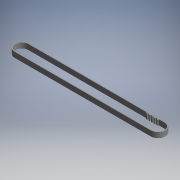
# Autodesk Inventor part: HTBN600S5M-100_info-1-16-16
Saved by Autodesk Inventor 2017.3 (Build 213256000, 256)
## iProperties
Part Number: HTBN600S5M-100_info-1-16-16
Material: Generic
Catalog Web Link: www.cadenas.de
Description: HTBN__S5M-High TorqueTiming Belts S5M (Pitch 5mm)
Vendor: MISUMI
Document SubType Name: Modeling
Designer: partserver
Manufacturer: MISUMI
Mass: 9.29796 g
Surface Area: 140.356 cm^2
Volume: 9.29796 cm^3
Density: 1 g/cm^3
Appearance: PSOLRGB-175-175-175
Category: PARTsolutions
Company: MISUMI
Title: HTBN600S5M-100
Author: Cadenas PARTsolutions
Comments: High TorqueTiming Belts S5M (Pitch 5mm)
PSOL_IDENT_0: {$CADENAS_DATA\23d-libs\misumi\metric\48_timing_belts\htbn_s5m.prj},209 {VTYP=3D},{NB=HTBN600S5M-100
PSOL_IDENT_1: _info-1-16-16},{LINA=HTBN600S5M-100},{NN=HTBN__S5M},{DATE=30.10.2020 16:17:07},{GEOMDATE=07.05.2015
PSOL_IDENT_2: 08:08:01},{VERSION=},{LINEID=10},{WBVAR=NT,RSSP,NT1,NT2},{WBNUMERIC=NT,NT1,NT2}  {NB=HTBN600S5M-100_
PSOL_IDENT_3: info-1-16-16},{LINA=HTBN600S5M-100},{KT=DUMMY},{PN=HTBN600S5M-100},{MATBR=Chloroprene Rubber},{MATTR=
PSOL_IDENT_4: Chloroprene Rubber},{MATCW=Glass Fiber Cord},{MATBC=Nylon Cloth},{OT=-30~90},{BNO=600S5M},{BNW=10},{
PSOL_IDENT_5: NT=120},{BC=600},{PITCH=5},{RAA=3.25},{LRR=3.25},{H=3.41},{HH=1.91},{II=1.5},{PLD=0.480},{BNWALG=100
PSOL_IDENT_6: },{TS=HTBN},{RSSP=1},{RSSP1= '1','900 or Less','2','Over 900, 1200 or Less','3','Over 1200, 1800 or
PSOL_IDENT_7: Less','4','Over 1800, 3600 or Less','5','Over 3600, 4800 or Less','6','Over 4800, 10000 or Less' },{
PSOL_IDENT_8: NT1=16},{NT2=16},{NT1A=16,18,19,20,22,24,25,26,28,30,32,34,36,40,44,48,50,60},{NT1A0=16,18,19,20,22,
PSOL_IDENT_9: 24,25,26,28,30,32,34,36,40,44,48,50,60},{NT1A1=0},{NT2A=16,18,19,20,22,24,25,26,28,30,32,34,36,40,44
PSOL_IDENT_10: ,48,50,60,72},{DRIVEP=25.46479},{DRIVENP=25.46479},{DRP=24.504791},{DRNP=24.504791},{C=260.00},{BB=1
PSOL_IDENT_11: 040.00000},{NOTE=-},{ASSCFGC=NT2,C},{ASSCFGCNOTE=-},{FS=32.00},{FL=32.00},{NT1SCR=16,18,19,20,22,24,
PSOL_IDENT_12: 25,26,28,30,32,34,36,40,44,48,50,60},{NT2SCR=16,18,19,20,22,24,25,26,28,30,32,34,36,40,44,48,50,60,7
PSOL_IDENT_13: 2}
NB: HTBN600S5M-100_info-1-16-16
NN: HTBN__S5M
NT: 120
NBSYN: $PN._info-$RSSP.-$NT1.-$NT2.
LINA: HTBN600S5M-100
CATALOG: Misumi
PN: HTBN600S5M-100
MATBR: Chloroprene Rubber
MATTR: Chloroprene Rubber
MATCW: Glass Fiber Cord
MATBC: Nylon Cloth
OT: -30~90
BNO: 600S5M
BNW: 10
BC: 600
PITCH: 5
RAA: 3.25
LRR: 3.25
H: 3.41
HH: 1.91
II: 1.5
PLD: 0.48
RSSP: 900 or Less
NT1: 16
NT2: 16
C: 260
NOTE: -
SUPPLIER: MISUMI
ARTICLENO: HTBN600S5M-100_info-1-16-16
BOMINFO: HTBN600S5M-100
CREATOR: CADENAS GmbH
Autodesk Inventor part; units mm, degrees
sketch "Sketch_1" plane through (0, 0, 0) normal (0, 0, 1) x (1, 0, 0)
  line L0 (10, 12.2524) -> (10.875, 12.2524)
  arc A0 (10.875, 12.2524) -> (11.4955, 10.3424) centre (14.125, 12.2524) ccw
  line L1 (11.4955, 10.3424) -> (13.5045, 10.3424)
  arc A1 (13.5045, 10.3424) -> (14.125, 12.2524) centre (10.875, 12.2524) ccw
  line L2 (14.125, 12.2524) -> (15.875, 12.2524)
  arc A2 (15.875, 12.2524) -> (16.4955, 10.3424) centre (19.125, 12.2524) ccw
  line L3 (16.4955, 10.3424) -> (18.5045, 10.3424)
  arc A3 (18.5045, 10.3424) -> (19.125, 12.2524) centre (15.875, 12.2524) ccw
  line L4 (19.125, 12.2524) -> (20.875, 12.2524)
  arc A4 (20.875, 12.2524) -> (21.4955, 10.3424) centre (24.125, 12.2524) ccw
  line L5 (21.4955, 10.3424) -> (23.5045, 10.3424)
  arc A5 (23.5045, 10.3424) -> (24.125, 12.2524) centre (20.875, 12.2524) ccw
  line L6 (24.125, 12.2524) -> (25.875, 12.2524)
  arc A6 (25.875, 12.2524) -> (26.4955, 10.3424) centre (29.125, 12.2524) ccw
  line L7 (26.4955, 10.3424) -> (28.5045, 10.3424)
  arc A7 (28.5045, 10.3424) -> (29.125, 12.2524) centre (25.875, 12.2524) ccw
  line L8 (29.125, 12.2524) -> (30.875, 12.2524)
  arc A8 (30.875, 12.2524) -> (31.4955, 10.3424) centre (34.125, 12.2524) ccw
  line L9 (31.4955, 10.3424) -> (33.5045, 10.3424)
  arc A9 (33.5045, 10.3424) -> (34.125, 12.2524) centre (30.875, 12.2524) ccw
  line L10 (34.125, 12.2524) -> (35, 12.2524)
  line L11 (35, 12.2524) -> (35, 13.7524)
  line L12 (35, 13.7524) -> (10, 13.7524)
  line L13 (10, 13.7524) -> (10, 12.2524)
  constraints: 28 end point, 20 point on circle, 10 centre point
extrude "Extrusion1" add sketch "Sketch_1" along normal mid plane 10
sketch "Sketch_2" plane through (0, 0, 0) normal (0, 0, 1) x (1, 0, 0)
  arc A0 (0, 13.7524) -> (0, -13.7524) centre (0, 0) ccw
  line L0 (0, -13.7524) -> (260, -13.7524)
  arc A1 (260, -13.7524) -> (260, 13.7524) centre (260, 0) ccw
  line L1 (260, 13.7524) -> (0, 13.7524)
  arc A2 (0, 12.2524) -> (0, -12.2524) centre (0, 0) ccw
  line L2 (0, -12.2524) -> (260, -12.2524)
  arc A3 (260, -12.2524) -> (260, 12.2524) centre (260, 0) ccw
  line L3 (260, 12.2524) -> (0, 12.2524)
  constraints: 8 end point, 8 point on circle, 4 centre point
extrude "Extrusion2" add sketch "Sketch_2" along normal mid plane 10
ref_plane "C1_XY" through (0, 0, 0) normal (0, 0, 1) x (1, 0, 0)
ref_plane "C1_YZ" through (0, 0, 0) normal (1, 0, 0) x (0, 1, 0)
ref_plane "C1_ZX" through (0, 0, 0) normal (0, 1, 0) x (0, 0, 1)
body "Solid1"
